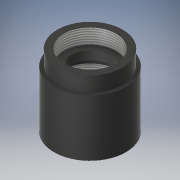
# Autodesk Inventor part: holder2
Saved by Autodesk Inventor 2017 (Build 210142000, 142)
## iProperties
Created: 2016-06-16
Part Number: holder2
Material: Generic
Document SubType Name: Modeling
Designer: Anna
Density: 1 g/cm^3
Appearance: Default
Author: Anna
Autodesk Inventor part; units mm, degrees
ref_plane "YZ Plane" through (0, 0, 0) normal (1, 0, 0) x (0, 1, 0)
ref_plane "XZ Plane" through (0, 0, 0) normal (0, 1, 0) x (-1, 0, 0)
ref_plane "XY Plane" through (0, 0, 0) normal (0, 0, 1) x (1, 0, 0)
sketch "Sketch1" plane through (0, 0, 0) normal (0, 1, 0) x (-1, 0, 0)
  circle A0 centre (0, 0) radius 6
  circle A1 centre (0, 0) radius 7.5
  dimension "d0" = 12
  dimension "d1" = 15
  constraints: 2 centre point, 2 coincident
  measures "d0" diameter of A0
  measures "d1" diameter of A1
extrude "Extrusion1" add sketch "Sketch1" along normal blind 3.5
sketch "Sketch2" plane through (0, 0, 0) normal (0, -1, 0) x (1, 0, 0)
  circle A0 centre (0, 0) radius 4.5
  circle A1 centre (0, 0) radius 8.25
  dimension "d4" = 9
  dimension "d5" = 16.5
  constraints: 2 centre point, 2 coincident
  measures "d4" diameter of A0
  measures "d5" diameter of A1
extrude "Extrusion2" add sketch "Sketch2" along normal blind 2
sketch "Sketch3" plane through (0, -2, 0) normal (0, -1, 0) x (1, 0, 0)
  circle A0 centre (0, 0) radius 6.75
  circle A1 centre (0, 0) radius 8.25 projected
  circle A2 centre (0, 0) radius 8.25
  dimension "d8" = 13.5
  dimension "d9" = 16.5
  constraints: 2 centre point, 2 coincident
  measures "d8" diameter of A0
  measures "d9" diameter of A2
extrude "Extrusion3" add sketch "Sketch3" along normal blind 11
sketch "Sketch4" plane through (0, -13, 0) normal (0, -1, 0) x (1, 0, 0)
  point P0 (0, 0)
sketch "Sketch9" plane through (0, -2, 0) normal (0, -1, 0) x (1, 0, 0)
  circle A0 centre (0, 0) radius 6.45
  circle A1 centre (0, 0) radius 6.75
  dimension "d54" = 12.9
  dimension "d55" = 13.5
  constraints: 2 centre point, 2 coincident
  measures "d54" diameter of A0
  measures "d55" diameter of A1
extrude "Extrusion4" add sketch "Sketch9" along normal blind 2
thread "Thread4" size "M12x0.5" class "6H" standard "ISO Metric profile" full length
thread "Thread5" size "M14x0.5" class "6H" standard "ISO Metric profile" length 9
equation "\"d25\" = 60deg"
equation "\"Sketch5_Pitch\" = 0.5"
equation "\"d43\" = 60deg"
equation "\"Sketch7_Pitch\" = 0.5"
body "Solid1"
